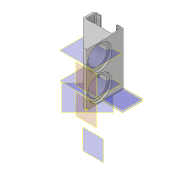
# Autodesk Inventor part: 30_Cube_Insert_Filter_Revolver_Filter_base_twin
Saved by Autodesk Inventor 2022 (Build 260153000, 153)
## iProperties
Created: 2021-09-13
Part Number: 30_Cube_Insert_Filter_Revolver_Filter_base_twin
Material: Generic
Document SubType Name: Modeling
Designer: diederichbenedict
Density: 1 g/cm^3
Appearance: Default
Mass: 6.97028 g
Surface Area: 48.8121 cm^2
Volume: 6.97028 cm^3
Author: diederichbenedict
Autodesk Inventor part; units mm, degrees
ref_plane "YZ Plane" through (0, 0, 0) normal (1, 0, 0) x (0, 1, 0)
ref_plane "XZ Plane" through (0, 0, 0) normal (0, 1, 0) x (-1, 0, 0)
ref_plane "XY Plane" through (0, 0, 0) normal (0, 0, 1) x (1, 0, 0)
ref_plane "Work Plane1" through (-34.3358, -34.38, 2.0699) normal (0, -1, 0) x (0.7071068, 0, -0.7071068)
ref_plane "Work Plane4" through (-9.5871, -34.38, 28.2329) normal (0, -1, 0) x (1, 0, 0)
ref_plane "Work Plane3" through (-9.5871, -32.38, 28.2329) normal (0, -1, 0) x (1, 0, 0)
sketch "Sketch1" plane through (-9.5871, -34.38, 28.2329) normal (0, -1, 0) x (1, 0, 0)
  line L0 (0.7071, -1.3185) -> (0.7071, -26.3185) construction
  line L1 (0.7071, -1.3185) -> (1.7071, -1.3185) construction
  line L2 (0.7071, -26.3185) -> (1.7071, -26.3185) construction
  line L3 (-4.2929, -0.7071) -> (-31.7929, -28.2071)
  line L4 (-31.7929, -28.2071) -> (0.7071, -28.2071)
  line L5 (0.7071, -28.2071) -> (0.7071, -0.7071)
  line L6 (0.7071, -0.7071) -> (-4.2929, -0.7071)
  line L7 (-4.2929, -0.7071) -> (-4.2929, -28.2071)
  line L8 (-4.2929, -28.2071) -> (0.7071, -28.2071)
  line L9 (0.7071, -0.7071) -> (3.5978, -0.7071)
  line L10 (2.5336, 1.8671) -> (2.3871, 1.8671) projected
  line L11 (0.7071, -0.7071) -> (0.7071, -28.2071)
  line L12 (0.7071, -28.2071) -> (-31.7929, -28.2071)
  point P0 (9.5871, -28.2329)
  dimension "d1" = 5
  dimension "d96" = 27.5
  dimension "d97" = 135
  constraints: 22 end point, 4 perpendicular, 3 horizontal, 2 point on line, 1 collinear, 2 other
  measures "d1" distance of L5.end L3.start
  measures "d96" distance between parallel lines of L4 L6
  measures "d97" angle of L7 L3
extrude "Extrusion1" add sketch "Sketch1" against normal blind 28
ref_plane "Work Plane5" through (-9.5871, -20.38, 28.2329) normal (0, -1, 0) x (1, 0, 0)
ref_plane "Work Plane6" through (-11.0013, -34.38, 27.5258) normal (0, 0, 1) x (1, 0, 0)
sketch "Sketch4" plane through (-8.88, -34.38, 27.5258) normal (-1, 0, 0) x (0, 0, 1)
  line L0 (0, 0) -> (-27.5, 0) projected
  line L1 (-27.5, 28) -> (0, 28) projected
  circle A0 centre (-13.75, 14) radius 10
  line L2 (0, 0) -> (0, 28) projected
  point P0 (-27.5258, 34.38)
  dimension "d89" = 28
  dimension "d90" = 20
  dimension "d91" = 14
  dimension "d98" = 13.75
  constraints: 1 centre point
  measures "d89" distance between parallel lines of L0 L1
  measures "d90" diameter of A0
  measures "d91" distance from line of A0.centre L0
  measures "d98" distance from line of A0.centre L2
extrude "Extrusion4" cut sketch "Sketch4" along normal through all
sketch "Sketch9" plane through (-11.38, -34.38, 30.0258) normal (-0.7071068, 0, 0.7071068) x (0.7071068, 0, 0.7071068)
  ellipse E0 centre (-22.981, 14) end of major axis (-37.1231, 14) minor radius 10 projected
  circle A0 centre (-22.981, 14) radius 12.75
  point P0 (-13.1846, 34.38)
  dimension "d99" = 25.5
  constraints: 1 centre point, 1 coincident, 1 other
  measures "d99" diameter of A0
extrude "Extrusion9" cut sketch "Sketch9" against normal blind 3.3 contours A0 E0 | E0 A0 | A0 E0 picked at (-31.5654, 13.4232) picked at (-24.148, 3.1781) picked at (-21.814, 24.8219)
sketch "Sketch3" plane through (-8.88, -34.38, 27.5258) normal (-1, 0, 0) x (0, 0, 1)
  circle A0 centre (-13.75, 14) radius 10 projected
  circle A1 centre (-13.75, 14) radius 13
  point P0 (-27.5258, 34.38)
  point P1 (13.1114, 14)
  dimension "d100" = 26
  constraints: 1 centre point, 1 coincident
  measures "d100" diameter of A1
extrude "Extrusion3" cut sketch "Sketch3" along normal blind 4 contours A0 | A1
sketch "Sketch13" plane through (-12.38, -34.38, 29.0258) normal (-0.7071068, 0, 0.7071068) x (0.7071068, 0, 0.7071068)
  arc A0 (-10.3808, 20.1186) -> (-32.7527, 20.1186) centre (-21.5668, 14) ccw projected
  circle A1 centre (-7.0668, 22.5) radius 1.4
  circle A2 centre (-7.0668, 5.5) radius 1.4
  circle A3 centre (-36.0668, 14) radius 1.4
  point P0 (-11.7703, 34.38)
  point P1 (-18.5424, 14)
  dimension "d101" = 2.8
  dimension "d102" = 2.8
  dimension "d103" = 14.5
  dimension "d104" = 14.5
  dimension "d105" = 14.5
  dimension "d106" = 2.8
  constraints: 3 centre point
  measures "d101" diameter of A2
  measures "d102" diameter of A3
  measures "d103" horizontal distance of A1.centre A0.centre
  measures "d104" horizontal distance of A0.centre A2.centre
  measures "d105" distance of A0.centre A3.centre
  measures "d106" diameter of A1
extrude "Extrusion13" cut sketch "Sketch13" against normal blind 10
pattern_linear "Rectangular Pattern1" count 2 spacing 28 along (0, 1, 0) of "Extrusion1", "Extrusion4", "Extrusion9", "Extrusion3", "Extrusion13" first direction both ways yes
ref_plane "Arbeitsebene13" through (-3.6065, -62.7242, 27.5258) normal (0, 0, -1) x (-1, 0, 0)
sketch "Sketch16" plane through (-8.88, -62.38, 27.5258) normal (0, 0, 1) x (1, 0, 0)
  ellipse E0 centre (-13.3299, 42) end of major axis (-13.3299, 54.75) minor radius 9.0156 projected
  circle A0 centre (-13.3299, 42) radius 1.5708
  point P0 (8.88, 62.38)
  constraints: 1 centre point, 1 coincident, 1 other
extrude "Extrusion15" cut sketch "Sketch16" against normal through all contours A0
sketch "Skizze20" plane through (-13.88, -34.38, 0.0258) normal (0, -1, 0) x (1, 0, 0)
  circle A0 centre (27.7649, 33.0797) radius 1.45
  point P0 (13.88, -0.0258)
  dimension "d93" = 2.9
  constraints: 1 centre point
  measures "d93" diameter of A0
extrude "Extrusion17" cut sketch "Skizze20" against normal blind 10
sketch "Skizze22" plane through (-13.88, -34.38, 27.5258) normal (0, -1, 0) x (1, 0, 0)
  arc A0 (-24.0858, -24.0858) -> (-22.6716, -27.5) centre (-22.6716, -25.5) ccw projected
  line L0 (-22.6716, -27.5) -> (5, -27.5) projected
  line L1 (5, -27.5) -> (5, 0) projected
  line L2 (5, 0) -> (0, 0) projected
  line L3 (0, 0) -> (-24.0858, -24.0858) projected
  line L4 (1.5971, -37.3) -> (1.5971, -29.5) projected
  line L5 (1.5971, -29.5) -> (0.3971, -28.3) projected
  line L6 (0.3971, -28.3) -> (-23.6029, -28.3) projected
  line L7 (-23.6029, -28.3) -> (-24.8029, -29.5) projected
  line L8 (-24.8029, -29.5) -> (-24.8029, -37.3) projected
  line L9 (-24.8029, -37.3) -> (-24.2029, -37.9) projected
  line L10 (-24.2029, -37.9) -> (-17.6029, -37.9) projected
  line L11 (-17.6029, -37.9) -> (-17.6029, -36.7579) projected
  arc A1 (-17.4477, -36.5266) -> (-17.6029, -36.7579) centre (-17.3529, -36.7579) ccw projected
  arc A2 (-17.4477, -36.5266) -> (-16.8701, -36.0273) centre (-17.9029, -35.4163) ccw projected
  arc A3 (-16.6767, -35.9055) -> (-16.8701, -36.0273) centre (-16.6549, -36.1546) ccw projected
  line L12 (-16.6767, -35.9055) -> (-16.3311, -35.8753) projected
  arc A4 (-16.3311, -35.8753) -> (-16.1029, -35.6262) centre (-16.3529, -35.6262) ccw projected
  line L13 (-16.1029, -35.6262) -> (-16.1029, -35.1738) projected
  arc A5 (-16.1029, -35.1738) -> (-16.3311, -34.9248) centre (-16.3529, -35.1738) ccw projected
  line L14 (-16.3311, -34.9248) -> (-16.6976, -34.8927) projected
  arc A6 (-16.8874, -34.7768) -> (-16.6976, -34.8927) centre (-16.6758, -34.6436) ccw projected
  arc A7 (-16.8874, -34.7768) -> (-17.4477, -34.3059) centre (-17.9029, -35.4163) ccw projected
  arc A8 (-17.6029, -34.0746) -> (-17.4477, -34.3059) centre (-17.3529, -34.0746) ccw projected
  line L15 (-17.6029, -34.0746) -> (-17.6029, -33.4) projected
  line L16 (-17.6029, -33.4) -> (-17.1029, -32.9) projected
  line L17 (-17.1029, -32.9) -> (-6.1029, -32.9) projected
  line L18 (-6.1029, -32.9) -> (-5.6029, -33.4) projected
  line L19 (-5.6029, -33.4) -> (-5.6029, -34.0746) projected
  arc A9 (-5.758, -34.3059) -> (-5.6029, -34.0746) centre (-5.8529, -34.0746) ccw projected
  arc A10 (-5.758, -34.3059) -> (-6.3183, -34.7768) centre (-5.3029, -35.4163) ccw projected
  arc A11 (-6.5081, -34.8927) -> (-6.3183, -34.7768) centre (-6.5299, -34.6436) ccw projected
  line L20 (-6.5081, -34.8927) -> (-6.8747, -34.9248) projected
  arc A12 (-6.8747, -34.9248) -> (-7.1029, -35.1738) centre (-6.8529, -35.1738) ccw projected
  line L21 (-7.1029, -35.1738) -> (-7.1029, -35.6262) projected
  arc A13 (-7.1029, -35.6262) -> (-6.8747, -35.8753) centre (-6.8529, -35.6262) ccw projected
  line L22 (-6.8747, -35.8753) -> (-6.529, -35.9055) projected
  arc A14 (-6.3357, -36.0273) -> (-6.529, -35.9055) centre (-6.5508, -36.1546) ccw projected
  arc A15 (-6.3357, -36.0273) -> (-5.758, -36.5266) centre (-5.3029, -35.4163) ccw projected
  arc A16 (-5.6029, -36.7579) -> (-5.758, -36.5266) centre (-5.8529, -36.7579) ccw projected
  line L23 (-5.6029, -36.7579) -> (-5.6029, -37.9) projected
  line L24 (-5.6029, -37.9) -> (0.9971, -37.9) projected
  line L25 (0.9971, -37.9) -> (1.5971, -37.3) projected
  circle A17 centre (-4.7029, -30.895) radius 2.1 projected
  circle A18 centre (-18.5029, -30.895) radius 2.1 projected
  line L26 (-23.6029, -28.3) -> (-24.8029, -29.5) projected
  arc A19 (-17.4477, -36.5266) -> (-16.8701, -36.0273) centre (-17.9029, -35.4162) ccw projected
  arc A20 (-16.6767, -35.9055) -> (-16.8701, -36.0273) centre (-16.6549, -36.1546) ccw projected
  line L27 (-16.6767, -35.9055) -> (-16.3311, -35.8753) projected
  arc A21 (-16.3311, -35.8753) -> (-16.1029, -35.6262) centre (-16.3529, -35.6262) ccw projected
  line L28 (-16.1029, -35.6262) -> (-16.1029, -35.1738) projected
  arc A22 (-16.1029, -35.1738) -> (-16.3311, -34.9247) centre (-16.3529, -35.1738) ccw projected
  line L29 (-16.3311, -34.9247) -> (-16.6976, -34.8927) projected
  arc A23 (-16.8874, -34.7768) -> (-16.6976, -34.8927) centre (-16.6758, -34.6436) ccw projected
  arc A24 (-16.8874, -34.7768) -> (-17.4477, -34.3059) centre (-17.9029, -35.4162) ccw projected
  arc A25 (-17.6029, -34.0746) -> (-17.4477, -34.3059) centre (-17.3529, -34.0746) ccw projected
  line L30 (-17.6029, -34.0746) -> (-17.6029, -33.4) projected
  line L31 (-17.6029, -33.4) -> (-17.1029, -32.9) projected
  line L32 (-17.1029, -32.9) -> (-6.1029, -32.9) projected
  line L33 (-6.1029, -32.9) -> (-5.6029, -33.4) projected
  line L34 (-5.6029, -33.4) -> (-5.6029, -34.0746) projected
  arc A26 (-5.758, -34.3059) -> (-5.6029, -34.0746) centre (-5.8529, -34.0746) ccw projected
  arc A27 (-5.758, -34.3059) -> (-6.3183, -34.7768) centre (-5.3029, -35.4162) ccw projected
  arc A28 (-6.5081, -34.8927) -> (-6.3183, -34.7768) centre (-6.5299, -34.6436) ccw projected
  line L35 (-6.5081, -34.8927) -> (-6.8747, -34.9247) projected
  arc A29 (-6.8747, -34.9247) -> (-7.1029, -35.1738) centre (-6.8529, -35.1738) ccw projected
  line L36 (-7.1029, -35.1738) -> (-7.1029, -35.6262) projected
  arc A30 (-7.1029, -35.6262) -> (-6.8747, -35.8753) centre (-6.8529, -35.6262) ccw projected
  line L37 (-6.8747, -35.8753) -> (-6.529, -35.9055) projected
  arc A31 (-6.3357, -36.0273) -> (-6.529, -35.9055) centre (-6.5508, -36.1546) ccw projected
  arc A32 (-6.3357, -36.0273) -> (-5.758, -36.5266) centre (-5.3029, -35.4162) ccw projected
  arc A33 (-5.6029, -36.7579) -> (-5.758, -36.5266) centre (-5.8529, -36.7579) ccw projected
  line L38 (-5.6029, -36.7579) -> (-5.6029, -37.9) projected
  line L39 (-5.6029, -37.9) -> (1.2971, -37.9) projected
  line L40 (1.2971, -37.9) -> (1.8971, -37.3) projected
  line L41 (1.8971, -37.3) -> (1.8971, -33.9) projected
  arc A34 (1.8971, -33.1) -> (1.8971, -33.9) centre (2.1971, -33.5) ccw projected
  line L42 (1.8971, -33.1) -> (1.8971, -28.5) projected
  line L43 (1.8971, -28.5) -> (1.2971, -27.9) projected
  line L44 (1.2971, -27.9) -> (-5.2029, -27.9) projected
  line L45 (-5.2029, -27.9) -> (-5.6029, -28.3) projected
  line L46 (-5.6029, -28.3) -> (-17.6029, -28.3) projected
  line L47 (-17.6029, -28.3) -> (-18.0029, -27.9) projected
  line L48 (-18.0029, -27.9) -> (-24.5028, -27.9) projected
  line L49 (-24.5028, -27.9) -> (-25.1029, -28.5) projected
  line L50 (-25.1029, -28.5) -> (-25.1029, -37.3) projected
  line L51 (-25.1029, -37.3) -> (-24.5029, -37.9) projected
  line L52 (-24.5029, -37.9) -> (-17.6029, -37.9) projected
  line L53 (-17.6029, -37.9) -> (-17.6029, -36.7579) projected
  arc A35 (-17.4477, -36.5266) -> (-17.6029, -36.7579) centre (-17.3529, -36.7579) ccw projected
  line L54 (-24.565, -27.75) -> (-17.9407, -27.75)
  line L55 (-17.9407, -27.75) -> (-17.5407, -28.15)
  line L56 (-17.5407, -28.15) -> (-5.665, -28.15)
  line L57 (-5.665, -28.15) -> (-5.265, -27.75)
  line L58 (-5.265, -27.75) -> (1.3592, -27.75)
  line L59 (1.3592, -27.75) -> (2.0471, -28.4379)
  line L60 (2.0471, -28.4379) -> (2.0471, -33.1838)
  arc A36 (2.0471, -33.1838) -> (2.0471, -33.8162) centre (2.1971, -33.5) ccw
  line L61 (2.0471, -33.8162) -> (2.0471, -37.3621)
  line L62 (2.0471, -37.3621) -> (1.3593, -38.05)
  line L63 (1.3593, -38.05) -> (-5.7529, -38.05)
  line L64 (-5.7529, -38.05) -> (-5.7529, -36.7579)
  arc A37 (-5.7529, -36.7579) -> (-5.8149, -36.6654) centre (-5.8529, -36.7579) ccw
  arc A38 (-6.4648, -36.1036) -> (-5.8149, -36.6654) centre (-5.3029, -35.4162) ccw
  arc A39 (-6.4648, -36.1036) -> (-6.5421, -36.0549) centre (-6.5508, -36.1546) ccw
  line L65 (-6.5421, -36.0549) -> (-6.8877, -36.0247)
  arc A40 (-7.2529, -35.6262) -> (-6.8877, -36.0247) centre (-6.8529, -35.6262) ccw
  line L66 (-7.2529, -35.6262) -> (-7.2529, -35.1738)
  arc A41 (-6.8877, -34.7753) -> (-7.2529, -35.1738) centre (-6.8529, -35.1738) ccw
  line L67 (-6.8877, -34.7753) -> (-6.5212, -34.7432)
  arc A42 (-6.5212, -34.7432) -> (-6.4453, -34.6969) centre (-6.5299, -34.6436) ccw
  arc A43 (-5.8149, -34.1671) -> (-6.4453, -34.6969) centre (-5.3029, -35.4162) ccw
  arc A44 (-5.8149, -34.1671) -> (-5.7529, -34.0746) centre (-5.8529, -34.0746) ccw
  line L68 (-5.7529, -34.0746) -> (-5.7529, -33.4621)
  line L69 (-5.7529, -33.4621) -> (-6.165, -33.05)
  line L70 (-6.165, -33.05) -> (-17.0407, -33.05)
  line L71 (-17.0407, -33.05) -> (-17.4529, -33.4621)
  line L72 (-17.4529, -33.4621) -> (-17.4529, -34.0746)
  arc A45 (-17.4529, -34.0746) -> (-17.3908, -34.1671) centre (-17.3529, -34.0746) ccw
  arc A46 (-16.7605, -34.6969) -> (-17.3908, -34.1671) centre (-17.9029, -35.4162) ccw
  arc A47 (-16.7605, -34.6969) -> (-16.6846, -34.7432) centre (-16.6758, -34.6436) ccw
  line L73 (-16.6846, -34.7432) -> (-16.318, -34.7753)
  arc A48 (-15.9529, -35.1738) -> (-16.318, -34.7753) centre (-16.3529, -35.1738) ccw
  line L74 (-15.9529, -35.1738) -> (-15.9529, -35.6262)
  arc A49 (-16.318, -36.0247) -> (-15.9529, -35.6262) centre (-16.3529, -35.6262) ccw
  line L75 (-16.318, -36.0247) -> (-16.6636, -36.0549)
  arc A50 (-16.6636, -36.0549) -> (-16.741, -36.1036) centre (-16.6549, -36.1546) ccw
  arc A51 (-17.3908, -36.6654) -> (-16.741, -36.1036) centre (-17.9029, -35.4162) ccw
  arc A52 (-17.3908, -36.6654) -> (-17.4529, -36.7579) centre (-17.3529, -36.7579) ccw
  line L76 (-17.4529, -36.7579) -> (-17.4529, -38.05)
  line L77 (-17.4529, -38.05) -> (-24.565, -38.05)
  line L78 (-24.565, -38.05) -> (-25.2529, -37.3621)
  line L79 (-25.2529, -37.3621) -> (-25.2529, -28.4379)
  line L80 (-25.2529, -28.4379) -> (-24.565, -27.75)
  arc A53 (-24.0858, -24.0858) -> (-22.6716, -27.5) centre (-22.6716, -25.5) ccw projected
  line L81 (-24.0858, -24.0858) -> (-27.5, -27.5)
  line L82 (-27.5, -27.5) -> (-27.5, -39.05)
  line L83 (-27.5, -39.05) -> (-20.1967, -39.05)
  line L84 (-20.1967, -39.05) -> (-20.1967, -38.05)
  line L85 (5, -27.5) -> (5, -39.05)
  line L86 (5, -39.05) -> (-3.2022, -39.05)
  line L87 (-3.2022, -39.05) -> (-3.2022, -38.05)
  line L88 (-22.6716, -27.5) -> (-27.5, -27.5)
  point P0 (13.88, -27.5258)
  point P1 (5, -27.5)
  point P2 (-17.6029, -28.3)
  point P3 (-5.6029, -28.3)
  point P4 (-16.3311, -35.8753)
  point P5 (-16.1029, -35.1738)
  dimension "d114" = 0.15
  dimension "d115" = 1
  dimension "d116" = 1
  constraints: 70 end point, 34 point on circle, 17 centre point, 5 point on line, 4 perpendicular, 3 tangent, 1 coincident, 1 parallel, 1 vertical, 43 other
  measures "d114" distance between parallel lines of L48 L54
  measures "d115" distance between parallel lines of L77 L83
  measures "d116" distance between parallel lines of L63 L86
extrude "Extrusion18" add sketch "Skizze22" against normal up to surface (56 mm away) contours L0 L85 L86 L87 L63 L62 L61 A36 L60 L59 L58 L57 L56 L55 L54 L80 L79 L78 L77 L84 L83 L82 L88
chamfer "Fase2" distance 2 angle 45 2 edges at (-8.88, -6.38, -11.5242) (-41.38, -6.38, -11.5242)
sketch "Skizze23" plane through (-13.88, -34.38, 27.5258) normal (0, -1, 0) x (1, 0, 0)
  line L0 (-25.2529, -39.05) -> (-27.2529, -37.05) projected
  line L1 (-25.2529, -39.05) -> (-20.1967, -39.05) projected
  line L2 (-20.1967, -39.05) -> (-20.1967, -38.05) projected
  line L3 (-20.1967, -38.05) -> (-24.565, -38.05) projected
  line L4 (-24.565, -38.05) -> (-25.2529, -37.3621) projected
  line L5 (-25.2529, -37.3621) -> (-25.2529, -28.4379) projected
  line L6 (-25.2529, -28.4379) -> (-24.565, -27.75) projected
  line L7 (-24.565, -27.75) -> (-17.9407, -27.75) projected
  line L8 (-17.9407, -27.75) -> (-17.5407, -28.15) projected
  line L9 (-17.5407, -28.15) -> (-5.665, -28.15) projected
  line L10 (-5.665, -28.15) -> (-5.265, -27.75) projected
  line L11 (-5.265, -27.75) -> (1.3592, -27.75) projected
  line L12 (1.3592, -27.75) -> (2.0471, -28.4379) projected
  line L13 (2.0471, -28.4379) -> (2.0471, -33.1838) projected
  arc A0 (2.0471, -33.1838) -> (2.0471, -33.8162) centre (2.1971, -33.5) ccw projected
  line L14 (2.0471, -33.8162) -> (2.0471, -37.3621) projected
  line L15 (2.0471, -37.3621) -> (1.3593, -38.05) projected
  line L16 (1.3593, -38.05) -> (-3.2022, -38.05) projected
  line L17 (-3.2022, -38.05) -> (-3.2022, -39.05) projected
  line L18 (-3.2022, -39.05) -> (3, -39.05) projected
  line L19 (5, -37.05) -> (3, -39.05) projected
  line L20 (5, -37.05) -> (5, 0) projected
  line L21 (5, 0) -> (0, 0) projected
  line L22 (0, 0) -> (-27.2529, -27.2529) projected
  line L23 (-27.2529, -27.2529) -> (-27.2529, -37.05) projected
  line L24 (3, -39.05) -> (5, -37.05) projected
  line L25 (5.8412, 1.6556) -> (3.5, 1.6556)
  line L26 (3.5, 1.6556) -> (3.5, -38.55)
  line L27 (3.5, -38.55) -> (5.8412, -38.55)
  line L28 (5.8412, -38.55) -> (5.8412, 1.6556)
  point P0 (13.88, -27.5258)
  constraints: 8 end point, 2 parallel, 1 horizontal, 1 perpendicular, 1 point on line
extrude "Extrusion19" cut sketch "Skizze23" against normal through all contours L26 L25 L28 L27 L19 L20 L21 | L21 L20 L19 L26
ref_plane "Work Plane2" through (41.82, -7.88, -4) normal (0, -1, 0) x (1, 0, 0)
ref_plane "Work Plane7" through (-11.0013, -6.38, 27.5258) normal (0, 0, 1) x (1, 0, 0)
ref_plane "Work Plane9" through (-9.5871, 7.62, 28.2329) normal (0, -1, 0) x (1, 0, 0)
equation "\"d91\" = 0.5 * d89"
equation "\"d98\" = 0.5 * d96"
body "Solid1"
